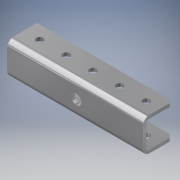
# Autodesk Inventor part: am-2222
Saved by Autodesk Inventor 2016 (Build 200138000, 138)
## iProperties
Category: Drive Base Kit
Company: Autodesk Inc.
Created: 2012-12-27
Part Number: am-2222
Material: Aluminum 6061
Document SubType Name: Modeling
Designer: Autodesk Inc.
Density: 1 g/cm^3
Catalog Web Link: www.andymark.com
Vendor: AndyMark Inc.
Appearance: Aluminum - Flat
Author: Autodesk Inc.
Autodesk Inventor part; units mm, degrees
ref_plane "YZ Plane" through (0, 0, 0) normal (1, 0, 0) x (0, 1, 0)
ref_plane "XZ Plane" through (0, 0, 0) normal (0, 1, 0) x (-1, 0, 0)
ref_plane "XY Plane" through (0, 0, 0) normal (0, 0, 1) x (1, 0, 0)
sketch "Sketch1" plane through (0, 0, 0) normal (0, 0, 1) x (1, 0, 0)
  line L0 (6.35, 28.575) -> (25.4, 28.575)
  line L1 (6.35, 31.75) -> (25.4, 31.75)
  line L2 (25.4, 0) -> (6.35, 0)
  arc A0 (0, 6.35) -> (6.35, 0) centre (6.35, 6.35) ccw
  line L3 (0, 6.35) -> (0, 25.4)
  arc A1 (6.35, 31.75) -> (0, 25.4) centre (6.35, 25.4) ccw
  line L4 (6.35, 31.75) -> (25.4, 31.75)
  line L5 (25.4, 28.575) -> (6.35, 28.575)
  arc A2 (6.35, 28.575) -> (3.175, 25.4) centre (6.35, 25.4) ccw
  line L6 (3.175, 25.4) -> (3.175, 6.35)
  arc A3 (3.175, 6.35) -> (6.35, 3.175) centre (6.35, 6.35) ccw
  line L7 (6.35, 3.175) -> (25.4, 3.175)
  line L8 (28.575, 3.175) -> (28.575, 0)
  line L9 (25.4, 31.75) -> (28.575, 31.75)
  line L10 (28.575, 28.575) -> (25.4, 28.575)
  line L11 (28.575, 31.75) -> (28.575, 28.575)
  line L12 (28.575, 0) -> (25.4, 0)
  line L13 (28.575, 3.175) -> (28.575, 0)
  line L14 (25.4, 3.175) -> (28.575, 3.175)
  point P0 (0, 0)
  constraints: 30 end point, 8 point on circle, 4 centre point
extrude "Extrusion1" add sketch "Sketch1" against normal blind 762
chamfer "Chamfer1" distance 3.175 angle 45 4 edges at (28.575, 30.1625, 0) (28.575, 1.5875, 0) (28.575, 30.1625, -762) (28.575, 1.5875, -762)
sketch "Sketch2" plane through (6.35, 31.75, 0) normal (0, 1, 0) x (1, 0, 0)
  line L0 (19.05, 0) -> (0, 0) projected
  line L1 (22.225, 3.175) -> (22.225, 758.825) projected
  point P0 (-6.35, 0)
  point P1 (9.525, 12.7)
  dimension "d5" = 12.7
  dimension "d6" = 12.7
  measures "d5" distance from line of point (9.525, 12.7) L0
  measures "d6" distance from line of point (9.525, 12.7) L1
hole "Hole1" at (15.875, 31.75, -12.7) direction (0, -1, 0) diameter 6.7056 end through all
pattern_linear "Rectangular Pattern1" count 30 spacing 25.4 along (0, 0, -1) of "Hole1"
sketch "Sketch3" plane through (0, 6.35, 0) normal (-1, 0, 0) x (0, 0, 1)
  line L0 (-0.2722, 19.0092) -> (-759.0056, 19.0092)
  line L1 (-759.0056, 19.0092) -> (-759.0056, 0.0408)
  line L2 (-0.2722, 0.0408) -> (-759.0056, 0.0408)
  line L3 (-0.2722, 0.0408) -> (-0.2722, 19.0092)
  circle A0 centre (-698.5852, 9.525) radius 4.78
  circle A1 centre (-111.2243, 9.525) radius 4.78
  circle A2 centre (-188.7416, 9.525) radius 3.6672
  circle A3 centre (-277.2605, 9.525) radius 3.6672
  circle A4 centre (-481.9921, 9.525) radius 3.6672
  circle A5 centre (-570.511, 9.525) radius 3.6672
  circle A6 centre (-469.3591, 9.525) radius 3.6672
  circle A7 centre (-583.1692, 9.525) radius 3.6672
  circle A8 centre (-289.9187, 9.525) radius 3.6672
  circle A9 centre (-176.1087, 9.525) radius 3.6672
  circle A10 centre (-551.6311, 9.525) radius 4.78
  circle A11 centre (-526.34, 9.525) radius 4.78
  circle A12 centre (-501.0489, 9.525) radius 4.78
  circle A13 centre (-258.2289, 9.525) radius 4.78
  circle A14 centre (-232.9378, 9.525) radius 4.78
  circle A15 centre (-207.6467, 9.525) radius 4.78
  circle A16 centre (-607.2589, 9.525) radius 1.5807
  circle A17 centre (-152.0189, 9.525) radius 1.5807
  circle A18 centre (-379.6389, 5.9842) radius 4.78
  circle A19 centre (-85.9332, 9.525) radius 4.78
  circle A20 centre (-673.294, 9.525) radius 4.78
  circle A21 centre (-648.0029, 9.525) radius 4.78
  circle A22 centre (-63.5, 9.525) radius 4.8006
  point P0 (0, -6.35)
  point P1 (-759.0056, -6.2819)
  dimension "d21" = 9.6012
  constraints: 23 centre point, 8 end point
  measures "d21" diameter of A22
extrude "Extrusion2" [suppressed]
sketch "Sketch4" plane through (6.35, 31.75, 0) normal (0, 1, 0) x (1, 0, 0)
  line L0 (-18.2452, 129.5546) -> (88.0083, 129.5546)
  line L1 (88.0083, 129.5546) -> (88.0083, 1027.7541)
  line L2 (88.0083, 1027.7541) -> (-18.2452, 1027.7541)
  line L3 (-18.2452, 1027.7541) -> (-18.2452, 129.5546)
  point P0 (-6.35, 0)
  constraints: 8 end point, 2 parallel, 1 horizontal, 1 perpendicular
extrude "Extrusion3" cut sketch "Sketch4" against normal blind 50.8
sketch "Sketch5" plane through (0, 6.35, 0) normal (-1, 0, 0) x (0, 0, 1)
  circle A0 centre (-63.5, 9.525) radius 4.8006
  dimension "d23" = 9.6012
  constraints: 1 centre point
  measures "d23" diameter of A0
extrude "Extrusion4" cut sketch "Sketch5" against normal through all
body "Solid1"
